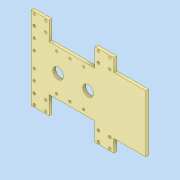
# Autodesk Inventor part: 底盘4.0
Saved by Autodesk Inventor 2019 (Build 230136000, 136)
## iProperties
Created: 2020-11-02
Part Number: 底盘4.0
Material: 尼龙 6/6
Document SubType Name: Modeling
Designer: Wang Hua
Density: 1.13 g/cm^3
Appearance: 尼龙 6
Mass: 59.1636 g
Surface Area: 303.115 cm^2
Volume: 52.3571 cm^3
Author: Wang Hua
Autodesk Inventor part; units mm, degrees
ref_plane "YZ Plane" through (0, 0, 0) normal (1, 0, 0) x (0, 1, 0)
ref_plane "XZ Plane" through (0, 0, 0) normal (0, 1, 0) x (-1, 0, 0)
ref_plane "XY Plane" through (0, 0, 0) normal (0, 0, 1) x (1, 0, 0)
sketch "草图1" plane through (0, 0, 0) normal (0, 0, 1) x (1, 0, 0)
  line L0 (-144.4444, 0) -> (-144.4444, 58)
  line L1 (-144.4444, 58) -> (-119.4444, 58)
  line L2 (-119.4444, 58) -> (-119.4444, 32)
  line L3 (-119.4444, 32) -> (-55.1944, 32)
  line L4 (-55.1944, 32) -> (-55.1944, 58)
  line L5 (-55.1944, 58) -> (-28.6944, 58)
  line L6 (-28.6944, 58) -> (-28.6944, 40)
  line L7 (-28.6944, 40) -> (16.3056, 40)
  line L8 (16.3056, 40) -> (16.3056, 0)
  line L9 (0, 0) -> (-166.6667, 0) construction
  line L10 (-144.4444, 0) -> (-144.4444, -58)
  line L11 (-144.4444, -58) -> (-119.4444, -58)
  line L12 (-119.4444, -58) -> (-119.4444, -32)
  line L13 (-119.4444, -32) -> (-55.1944, -32)
  line L14 (-55.1944, -32) -> (-55.1944, -58)
  line L15 (-55.1944, -58) -> (-28.6944, -58)
  line L16 (-28.6944, -58) -> (-28.6944, -40)
  line L17 (-28.6944, -40) -> (16.3056, -40)
  line L18 (16.3056, -40) -> (16.3056, 0)
  circle A0 centre (-106.5528, 0) radius 7.5
  circle A1 centre (-64.5976, 0) radius 7.5
  point P0 (-141.4444, -54)
  point P1 (-127.4444, -54)
  point P2 (-51.4444, -54)
  point P3 (-37.4444, -54)
  point P4 (-112.1204, -28)
  point P5 (-64.5976, -28)
  point P6 (-89.6514, -28)
  point P7 (-127.4444, -38)
  point P8 (-141.4444, -38)
  point P9 (-51.4444, -38)
  point P10 (-37.4444, -38)
  point P11 (-141.4444, 54)
  point P12 (-127.4444, 54)
  point P13 (-127.4444, 38)
  point P14 (-141.4444, 38)
  point P15 (-51.4444, 54)
  point P16 (-51.4444, 38)
  point P17 (-37.4444, 54)
  point P18 (-37.4444, 38)
  point P19 (-64.5976, 28)
  point P20 (-89.6514, 28)
  point P21 (-112.1204, 28)
  point P22 (-131.9444, 58)
  point P23 (-41.9444, 58)
  dimension "d0" = 25
  dimension "d1" = 26.5
  dimension "d3" = 32
  dimension "d4" = 40
  dimension "d5" = 45
  dimension "d6" = 58
  dimension "d7" = 15
  dimension "d8" = 15
  dimension "d29" = 28
  dimension "d30" = 28
  dimension "d31" = 28
  dimension "d36" = 90
  constraints: 38 end point, 19 symmetric about line, 7 perpendicular, 4 point on line, 2 centre point, 2 midpoint, 2 vertical, 1 collinear, 1 horizontal
  measures "d0" distance of L0.end L1.end
  measures "d1" distance of L4.end L5.end
  measures "d3" distance between parallel lines of L9 L3
  measures "d4" distance between parallel lines of L9 L7
  measures "d5" distance of L6.end L7.end
  measures "d6" distance of L0.start L0.end
  measures "d7" diameter of A0
  measures "d8" diameter of A1
  measures "d29" distance from line of L9 point (-112.12, 28)
  measures "d30" distance from line of L9 point (-89.651, 28)
  measures "d31" distance from line of L9 point (-64.598, 28)
  measures "d36" distance of point (-41.944, 58) point (-131.944, 58)
extrude "拉伸1" add sketch "草图1" along normal blind 4
sketch "草图2" plane through (0, 0, 4) normal (0, 0, 1) x (1, 0, 0)
  circle A0 centre (-64.5976, 0) radius 7.5 construction
  circle A1 centre (-106.5528, 0) radius 7.5 construction
  line L0 (-144.4444, -58) -> (-144.4444, 58) construction
  line L1 (-144.4444, 58) -> (-119.4444, 58) construction
  line L2 (-119.4444, 58) -> (-119.4444, 32) construction
  line L3 (-119.4444, 32) -> (-55.1944, 32) construction
  line L4 (-55.1944, 32) -> (-55.1944, 58) construction
  line L5 (-55.1944, 58) -> (-28.6944, 58) construction
  line L6 (-28.6944, 58) -> (-28.6944, 40) construction
  line L7 (-28.6944, 40) -> (16.3056, 40) construction
  line L8 (16.3056, 40) -> (16.3056, -40) construction
  line L9 (16.3056, -40) -> (-28.6944, -40) construction
  line L10 (-28.6944, -40) -> (-28.6944, -58) construction
  line L11 (-28.6944, -58) -> (-55.1944, -58) construction
  line L12 (-55.1944, -58) -> (-55.1944, -32) construction
  line L13 (-55.1944, -32) -> (-119.4444, -32) construction
  line L14 (-119.4444, -32) -> (-119.4444, -58) construction
  line L15 (-119.4444, -58) -> (-144.4444, -58) construction
  line L16 (-164.7255, 0) -> (-80.9793, 0) construction
  point P0 (0, 0)
  point P1 (-139.9444, 55)
  point P2 (-123.9444, 55)
  point P3 (-50.1944, 55)
  point P4 (-34.1944, 55)
  point P5 (-50.1944, 41)
  point P6 (-34.1944, 41)
  point P7 (-123.9444, 41)
  point P8 (-139.9444, 41)
  point P9 (-139.9444, -55)
  point P10 (-123.9444, -55)
  point P11 (-50.1944, -55)
  point P12 (-34.1944, -55)
  point P13 (-50.1944, -41)
  point P14 (-34.1944, -41)
  point P15 (-123.9444, -41)
  point P16 (-139.9444, -41)
  dimension "d32" = 3
  dimension "d33" = 3
  dimension "d34" = 16
  dimension "d37" = 4.5
  dimension "d38" = 14
  dimension "d39" = 4.5
  dimension "d40" = 14
  dimension "d41" = 4.5
  dimension "d42" = 16
  dimension "d43" = 16
  dimension "d44" = 14
  dimension "d45" = 3
  dimension "d46" = 5
  dimension "d47" = 5
  constraints: 8 symmetric about line, 2 end point, 1 horizontal
  measures "d32" distance from line of L1 point (-123.944, 55)
  measures "d33" distance from line of L1 point (-139.944, 55)
  measures "d34" distance of point (-123.944, 55) point (-139.944, 55)
  measures "d37" distance from line of L0 point (-139.944, 55)
  measures "d38" distance of point (-139.944, 55) point (-139.944, 41)
  measures "d39" distance from line of L0 point (-139.944, 41)
  measures "d40" distance of point (-123.944, 55) point (-123.944, 41)
  measures "d41" distance from line of L2 point (-123.944, 41)
  measures "d42" distance of point (-34.194, 55) point (-50.194, 55)
  measures "d43" distance of point (-34.194, 41) point (-50.194, 41)
  measures "d44" distance of point (-50.194, 55) point (-50.194, 41)
  measures "d45" distance from line of L5 point (-50.194, 55)
  measures "d46" distance from line of L4 point (-50.194, 41)
  measures "d47" distance from line of L4 point (-50.194, 55)
hole "孔2" at (-139.9444, 55, 4) at (-123.9444, 55, 4) at (-50.1944, 55, 4) at (-34.1944, 55, 4) at (-50.1944, 41, 4) at (-34.1944, 41, 4) at (-123.9444, 41, 4) at (-139.9444, 41, 4) at (-139.9444, -55, 4) at (-139.9444, -41, 4) at (-123.9444, -55, 4) at (-123.9444, -41, 4) at (-50.1944, -41, 4) at (-34.1944, -41, 4) at (-34.1944, -55, 4) at (-50.1944, -55, 4) direction (0, 0, -1) diameter 3.6 end through all
sketch "草图3" plane through (0, 0, 4) normal (0, 0, 1) x (1, 0, 0)
  circle A0 centre (-34.1944, -55) radius 1.8 construction
  circle A1 centre (-50.1944, -41) radius 1.8 construction
  circle A2 centre (-123.9444, -55) radius 1.8 construction
  circle A3 centre (-139.9444, -55) radius 1.8 construction
  circle A4 centre (-123.9444, 41) radius 1.8 construction
  circle A5 centre (-50.1944, 41) radius 1.8 construction
  circle A6 centre (-50.1944, 55) radius 1.8 construction
  circle A7 centre (-139.9444, 55) radius 1.8 construction
  circle A8 centre (-123.9444, 55) radius 1.8 construction
  circle A9 centre (-34.1944, 55) radius 1.8 construction
  circle A10 centre (-34.1944, 41) radius 1.8 construction
  circle A11 centre (-139.9444, 41) radius 1.8 construction
  circle A12 centre (-139.9444, -41) radius 1.8 construction
  circle A13 centre (-123.9444, -41) radius 1.8 construction
  circle A14 centre (-34.1944, -41) radius 1.8 construction
  circle A15 centre (-50.1944, -55) radius 1.8 construction
  circle A16 centre (-64.5976, 0) radius 7.5 construction
  circle A17 centre (-106.5528, 0) radius 7.5 construction
  line L0 (-144.4444, 58) -> (-144.4444, -58) construction
  line L1 (-144.4444, -58) -> (-119.4444, -58) construction
  line L2 (-119.4444, -58) -> (-119.4444, -32) construction
  line L3 (-119.4444, -32) -> (-55.1944, -32) construction
  line L4 (-55.1944, -32) -> (-55.1944, -58) construction
  line L5 (-55.1944, -58) -> (-28.6944, -58) construction
  line L6 (-28.6944, -58) -> (-28.6944, -40) construction
  line L7 (-28.6944, -40) -> (16.3056, -40) construction
  line L8 (16.3056, -40) -> (16.3056, 40) construction
  line L9 (16.3056, 40) -> (-28.6944, 40) construction
  line L10 (-28.6944, 40) -> (-28.6944, 58) construction
  line L11 (-28.6944, 58) -> (-55.1944, 58) construction
  line L12 (-55.1944, 58) -> (-55.1944, 32) construction
  line L13 (-55.1944, 32) -> (-119.4444, 32) construction
  line L14 (-119.4444, 32) -> (-119.4444, 58) construction
  line L15 (-119.4444, 58) -> (-144.4444, 58) construction
  line L16 (0, 0) -> (-184.5407, 0) construction
  point P0 (-139.9444, 25.8646)
  point P1 (-139.9444, 10.9473)
  point P2 (-108.7515, 25.8646)
  point P3 (-89.9847, 25.8646)
  point P4 (-70.7366, 25.8646)
  point P5 (-139.9444, -25.8646)
  point P6 (-139.9444, -10.9473)
  point P7 (-108.7515, -25.8646)
  point P8 (-89.9847, -25.8646)
  point P9 (-70.7366, -25.8646)
  constraints: 5 symmetric about line, 2 end point, 1 horizontal
hole "孔3" at (-139.9444, 25.8646, 4) at (-139.9444, 10.9473, 4) at (-108.7515, 25.8646, 4) at (-89.9847, 25.8646, 4) at (-70.7366, 25.8646, 4) at (-139.9444, -25.8646, 4) at (-139.9444, -10.9473, 4) at (-108.7515, -25.8646, 4) at (-89.9847, -25.8646, 4) at (-70.7366, -25.8646, 4) direction (0, 0, -1) diameter 3.2 end through all
